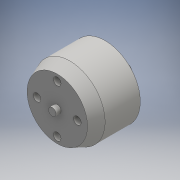
# Autodesk Inventor part: motor_generic
Saved by Autodesk Inventor 2016 (Build 200138000, 138)
## iProperties
Created: 2016-03-07
Part Number: motor_generic
Material: Generic
Document SubType Name: Modeling
Designer: dimas
Density: 1 g/cm^3
Appearance: Default
Author: dimas
Autodesk Inventor part; units mm, degrees
ref_plane "YZ Plane" through (0, 0, 0) normal (1, 0, 0) x (0, 1, 0)
ref_plane "XZ Plane" through (0, 0, 0) normal (0, 1, 0) x (-1, 0, 0)
ref_plane "XY Plane" through (0, 0, 0) normal (0, 0, 1) x (1, 0, 0)
sketch "Sketch1" plane through (0, 0, 0) normal (0, 1, 0) x (-1, 0, 0)
  circle A0 centre (0, 0) radius 14
  dimension "d0" = 28
  constraints: 1 centre point, 1 coincident
  measures "d0" diameter of A0
extrude "Extrusion1" add sketch "Sketch1" along normal blind 24
chamfer "Chamfer1" distance 2 distance2 5 1 edges at (14, 0, 0) measured on face at (13.5, 0, 0)
sketch "Sketch2" plane through (0, 0, 0) normal (0, -1, 0) x (1, 0, 0)
  circle A0 centre (0, 0) radius 9.5
  circle A1 centre (0, 0) radius 8
  line L0 (0, 0) -> (0, 9.5)
  line L1 (0, 0) -> (0, -9.5)
  line L2 (0, 0) -> (8, 0)
  line L3 (0, 0) -> (-8, 0)
  dimension "d6" = 19
  dimension "d7" = 16
  constraints: 8 end point, 4 point on circle, 2 centre point, 2 coincident, 2 point on line, 1 perpendicular, 1 vertical
  measures "d6" diameter of A0
  measures "d7" diameter of A1
hole "Hole1" at (0, 0, 9.5) at (-8, 0, 0) at (8, 0, 0) at (0, 0, -9.5) direction (0, 1, 0) diameter 3 depth 5 tip angle 118
chamfer "Chamfer2" distance 8 distance2 5 1 edges at (14, 24, 0) measured on face at (13.5, 24, 0)
sketch "Sketch3" plane through (0, 24, 0) normal (0, 1, 0) x (1, 0, 0)
  circle A0 centre (0, 0) radius 1.5
  dimension "d18" = 3
  constraints: 1 centre point, 1 coincident
  measures "d18" diameter of A0
extrude "Extrusion2" add sketch "Sketch3" along normal blind 4
sketch "Sketch4" plane through (0, 0, 0) normal (0, -1, 0) x (1, 0, 0)
  circle A0 centre (0, 0) radius 1.5
  dimension "d21" = 3
  constraints: 1 centre point, 1 coincident
  measures "d21" diameter of A0
extrude "Extrusion3" add sketch "Sketch4" along normal blind 2
body "Solid1"
